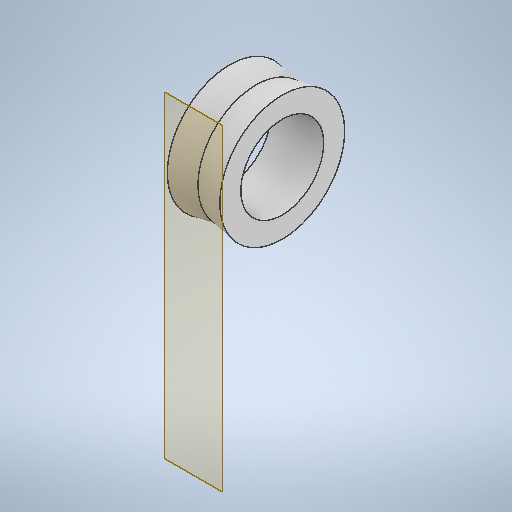
# Autodesk Inventor part: RUEDA
Saved by Autodesk Inventor 2025 (Build 290162000, 162)
## iProperties
Created: 2026-02-25
Part Number: RUEDA
Material: Caucho
Document SubType Name: Modeling
Designer: Frank
Density: 0.93 g/cm^3
Appearance: Valor por defecto
Author: Frank
Autodesk Inventor part; units mm, degrees
ref_plane "YZ Plane" through (0, 0, 0) normal (1, 0, 0) x (0, 1, 0)
ref_plane "XZ Plane" through (0, 0, 0) normal (0, 1, 0) x (-1, 0, 0)
sketch "Boceto1" plane through (0, 0, 0) normal (0, 0, 1) x (1, 0, 0)
  line L0 (-2.6681, 26.4223) -> (2.0819, 27.213)
  line L1 (2.0819, 27.213) -> (6.8319, 26.4223)
  line L2 (-2.6681, 26.4223) -> (-2.6681, 37.7223)
  line L3 (-2.6681, 37.7223) -> (6.8319, 37.7223)
  line L4 (6.8319, 37.7223) -> (6.8319, 26.4223)
  line L5 (-10.0441, 37.7223) -> (15.5042, 37.7223) construction
  dimension "d29" = 161.1
  dimension "d62" = 9.5
  dimension "d63" = 4.8153
  dimension "d65" = 4.8153
  dimension "d66" = 11.3
  constraints: 12 end point, 2 perpendicular, 1 horizontal, 1 vertical
  measures "d29" angle of L0 L1
  measures "d62" distance of L1.end L0.start
  measures "d63" distance of L0.end L1.end
  measures "d65" distance of L0.start L0.end
  measures "d66" distance of L0.start L2.end
revolve "Revolución1" add sketch "Boceto1" angle 360 about axis through (-10.0441, 37.7223, 0) along (1, 0, 0)
sketch "Boceto2" plane through (-2.6681, 37.7223, 0) normal (-1, 0, 0) x (0, 0, 1)
  circle A0 centre (0, 0) radius 7.5
  circle A1 centre (0, 0) radius 11.3 projected
  point P0 (0, -37.7223)
  dimension "d68" = 3.8
  constraints: 1 centre point, 1 coincident
  measures "d68" radial gap between concentric circles of A1 A0
extrude "Extrusión1" cut sketch "Boceto2" against normal through all contours A0
ref_plane "Plano de trabajo1" through (0, 0, 11.3) normal (0, 0, 1) x (1, 0, 0)
